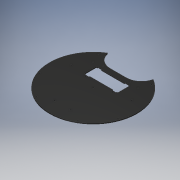
# Autodesk Inventor part: Hauptplatine
Saved by Autodesk Inventor 2018 (Build 220112000, 112)
## iProperties
Created: 2019-03-02
Part Number: Hauptplatine
Material: Kupfer
Document SubType Name: Modeling
Designer: RedBots
Density: 3.52371 g/cm^3
Appearance: Glänzend - schwarz
Mass: 200 g
Surface Area: 589.064 cm^2
Volume: 56.7583 cm^3
Author: RedBots
Autodesk Inventor part; units mm, degrees
ref_plane "YZ Plane" through (0, 0, 0) normal (1, 0, 0) x (0, 1, 0)
ref_plane "XZ Plane" through (0, 0, 0) normal (0, 1, 0) x (-1, 0, 0)
ref_plane "XY Plane" through (0, 0, 0) normal (0, 0, 1) x (1, 0, 0)
sketch "Skizze3" plane through (0, 0, 0) normal (0, 0, 1) x (1, 0, 0)
  arc A0 (-55.0029, 89.4409) -> (55.0029, 89.4409) centre (0, 0) ccw
  line L0 (0, 0) -> (55.0029, 89.4409) construction
  line L1 (0, 0) -> (105, 0) construction
  line L2 (0, 0) -> (-55.0029, 89.4409) construction
  line L3 (-55.0029, 89.4409) -> (-18.8829, 89.4409)
  line L4 (-18.8829, 89.4409) -> (-18.8829, 97.4409)
  arc A1 (-55.0029, 89.4409) -> (-18.8829, 60.4456) centre (-18.8829, 97.4409) ccw
  line L5 (55.0029, 89.4409) -> (18.8829, 89.4409)
  line L6 (18.8829, 89.4409) -> (18.8829, 97.4409)
  arc A2 (18.8839, 60.4456) -> (55.0029, 89.4409) centre (18.8829, 97.4409) ccw
  line L7 (18.8829, 97.4409) -> (18.8839, 60.4456) construction
  line L8 (18.8829, 97.4409) -> (55.0029, 89.4409) construction
  line L9 (-18.8829, 60.4456) -> (18.8839, 60.4456)
  line L10 (0, 0) -> (57.2785, 0) construction
  line L11 (0, 0) -> (57.2785, 0) construction
  line L12 (0, 0) -> (57.279, 0) construction
  line L13 (0, 0) -> (84.4383, 0) construction
  line L14 (0, 0) -> (90, 0) construction
  line L15 (0, 0) -> (90, 0) construction
  line L16 (0, 0) -> (90, 0) construction
  line L17 (0, 0) -> (97, 0) construction
  line L18 (0, 0) -> (97, 0) construction
  line L19 (0, 0) -> (97, 0) construction
  line L20 (0, 0) -> (97, 0) construction
  line L21 (0, 0) -> (100, 0) construction
  circle A3 centre (-93.9693, -34.202) radius 1.5
  line L22 (0, 0) -> (100, 0) construction
  line L23 (0, 0) -> (100, 0) construction
  line L24 (0, 0) -> (100, 0) construction
  circle A4 centre (-50, -86.6025) radius 1.5
  circle A5 centre (93.9693, -34.202) radius 1.5
  circle A6 centre (50, -86.6025) radius 1.5
  line L25 (0, 0) -> (100, 0) construction
  line L26 (0, 0) -> (100, 0) construction
  circle A7 centre (-64.2788, 76.6044) radius 1.5
  circle A8 centre (64.2788, 76.6044) radius 1.5
  line L27 (0, 0) -> (42, 0) construction
  line L28 (0, 0) -> (42, 0) construction
  circle A9 centre (-32.5, 56.2917) radius 1.5
  circle A10 centre (32.5, 56.2917) radius 1.5
  line L29 (-32.5, 56.2917) -> (32.5, 56.2917) construction
  line L30 (-32.5, 56.2917) -> (0, 0) construction
  line L31 (32.5, 56.2917) -> (0, 0) construction
  line L32 (0, 0) -> (0, -73.5) construction
  line L33 (0, -73.5) -> (-19, -73.5) construction
  circle A11 centre (-19, -73.5) radius 1.5
  line L34 (0, 0) -> (-64.2788, 76.6044) construction
  line L35 (0, 0) -> (100, 0) construction
  line L36 (0, 0) -> (64.2788, 76.6044) construction
  line L37 (0, 0) -> (100, 0) construction
  line L38 (0, 0) -> (-93.9693, -34.202) construction
  line L39 (0, 0) -> (100, 0) construction
  line L40 (0, 0) -> (93.9693, -34.202) construction
  line L41 (0, 0) -> (100, 0) construction
  line L42 (0, 0) -> (-50, -86.6025) construction
  line L43 (0, 0) -> (100, 0) construction
  line L44 (0, 0) -> (50, -86.6025) construction
  line L45 (0, 0) -> (100, 0) construction
  circle A12 centre (19, -73.5) radius 1.5
  line L46 (0, 0) -> (63.6529, 36.75) construction
  line L47 (0, 0) -> (73.5, 0) construction
  line L48 (63.6529, 36.75) -> (54.1529, 53.2045) construction
  circle A13 centre (54.1529, 53.2045) radius 1.5
  circle A14 centre (73.1529, 20.2955) radius 1.5
  circle A15 centre (-54.1529, 53.2045) radius 1.5
  circle A16 centre (-73.1529, 20.2955) radius 1.5
  circle A17 centre (0, 0) radius 1.5
  dimension "d22" = 105
  dimension "d23" = 58.41
  dimension "d24" = 63.18
  dimension "d25" = 36.12
  dimension "d26" = 8
  dimension "d27" = 90
  dimension "d28" = 36.12
  dimension "d29" = 8
  dimension "d30" = 90
  dimension "d31" = 77.51
  dimension "d140" = 3
  dimension "d153" = 65
  dimension "d154" = 120
  dimension "d163" = 60
  dimension "d172" = 73.5
  dimension "d173" = 19
  dimension "d174" = 100
  dimension "d175" = 130
  dimension "d176" = 100
  dimension "d177" = 50
  dimension "d178" = 100
  dimension "d179" = 160
  dimension "d180" = 100
  dimension "d181" = 20
  dimension "d182" = 100
  dimension "d183" = 120
  dimension "d184" = 100
  dimension "d185" = 60
  dimension "d186" = 73.5
  dimension "d187" = 30
  dimension "d188" = 19
  dimension "d189" = 3
  constraints: 59 end point, 58 horizontal, 17 centre point, 9 equal radius, 4 coincident, 4 perpendicular, 4 point on circle, 4 symmetric about line, 2 vertical, 1 horizontal alignment, 28 other
  measures "d23" angle of L1 L0
  measures "d24" angle of L0 L2
  measures "d25" distance of L2.end L3.end
  measures "d26" distance of L3.end L4.end
  measures "d27" angle of L4 L3
  measures "d28" distance of L0.end L5.end
  measures "d29" distance of L5.end L6.end
  measures "d30" angle of L5 L6
  measures "d31" angle of L7 L8
  measures "d140" diameter of A7
  measures "d153" distance of point (0, 0) L29.start
  measures "d154" angle of L11 L30
  measures "d163" angle of L10 L31
  measures "d173" distance of L32.end L33.end
  measures "d175" angle of L35 L34
  measures "d177" angle of L37 L36
  measures "d179" angle of L38 L39
  measures "d181" angle of L40 L41
  measures "d183" angle of L42 L43
  measures "d185" angle of L44 L45
  measures "d187" angle of L47 L46
  measures "d188" distance of L46.end L48.end
  measures "d189" diameter of A17
extrude "Extrusion3" add sketch "Skizze3" along normal blind 2
sketch "Skizze5" plane through (0, 0, 2) normal (0, 0, 1) x (1, 0, 0)
  line L0 (-40, 19.2917) -> (40, 19.2917)
  line L1 (40, 19.2917) -> (40, 47.2917)
  line L2 (40, 47.2917) -> (-40, 47.2917)
  line L3 (-40, 47.2917) -> (-40, 19.2917)
  line L4 (0, 0) -> (0, 47.2917) construction
  line L5 (-37.5, 47.2917) -> (-27.5, 47.2917)
  line L6 (-27.5, 47.2917) -> (-27.5, 49.2917)
  line L7 (-27.5, 49.2917) -> (-37.5, 49.2917)
  line L8 (-37.5, 49.2917) -> (-37.5, 47.2917)
  line L9 (-40, 33.2917) -> (40, 33.2917) construction
  line L10 (-37.5, 19.2917) -> (-27.5, 19.2917)
  line L11 (-27.5, 19.2917) -> (-27.5, 17.2917)
  line L12 (-27.5, 17.2917) -> (-37.5, 17.2917)
  line L13 (-37.5, 17.2917) -> (-37.5, 19.2917)
  line L14 (37.5, 47.2917) -> (27.5, 47.2917)
  line L15 (27.5, 47.2917) -> (27.5, 49.2917)
  line L16 (27.5, 49.2917) -> (37.5, 49.2917)
  line L17 (37.5, 49.2917) -> (37.5, 47.2917)
  line L18 (37.5, 19.2917) -> (27.5, 19.2917)
  line L19 (27.5, 19.2917) -> (27.5, 17.2917)
  line L20 (27.5, 17.2917) -> (37.5, 17.2917)
  line L21 (37.5, 17.2917) -> (37.5, 19.2917)
  circle A0 centre (-32.5, 14.2917) radius 1.5
  circle A1 centre (32.5, 14.2917) radius 1.5
  circle A2 centre (-32.5, 56.2917) radius 1.5 projected
  line L22 (-32.5, 49.2917) -> (-32.5, 56.2917) construction
  dimension "d158" = 80
  dimension "d159" = 28
  dimension "d164" = 10
  dimension "d165" = 2
  dimension "d169" = 3
  dimension "d171" = 7
  constraints: 46 end point, 13 symmetric about line, 4 midpoint, 4 parallel, 2 centre point, 2 horizontal, 2 perpendicular, 2 vertical, 1 point on line, 1 other
  measures "d158" distance of L2.end L1.end
  measures "d159" distance of L1.end L0.end
  measures "d164" distance of L7.end L6.end
  measures "d165" distance of L6.end L5.end
  measures "d169" distance from line of L12 A0.centre
  measures "d171" distance from line of L7 L22.end
extrude "Extrusion4" cut sketch "Skizze5" against normal up to next
